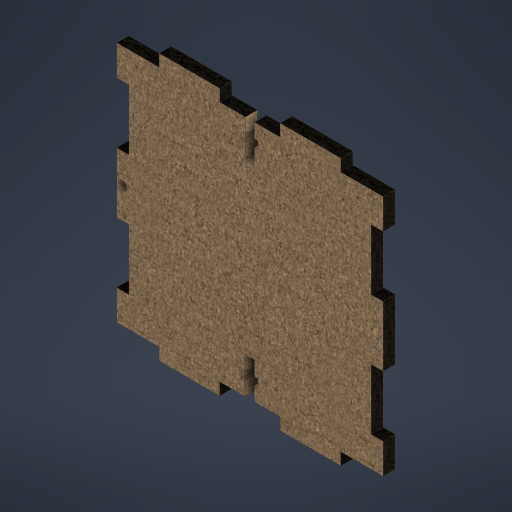
# Autodesk Inventor part: Car_Rear
Saved by Autodesk Inventor 2024.1 (Build 281209000, 209)
## iProperties
Created: 2023-08-04
Part Number: Car_Rear
Material: MDF Medium Density Fiberboard
Document SubType Name: Modeling
Designer: jaege
Density: 0.8 g/cm^3
Appearance: Cardboard - Corrugated
Author: jaege
Autodesk Inventor part; units mm, degrees
ref_plane "YZ Plane" through (0, 0, 0) normal (1, 0, 0) x (0, 1, 0)
ref_plane "XZ Plane" through (0, 0, 0) normal (0, 1, 0) x (-1, 0, 0)
ref_plane "XY Plane" through (0, 0, 0) normal (0, 0, 1) x (1, 0, 0)
sketch "Sketch1" plane through (0, 0, 0) normal (0, 0, 1) x (1, 0, 0)
  line L0 (70, 0) -> (80, 0) construction
  line L1 (80, 0) -> (80, 4) projected
  line L2 (70, 4) -> (80, 4) projected
  line L3 (70, 0) -> (70, 4) projected
  line L4 (50, 0) -> (70, 0) projected
  line L5 (30, 0) -> (50, 0) construction
  line L6 (50, 0) -> (50, 4) projected
  line L7 (30, 4) -> (50, 4) projected
  line L8 (30, 0) -> (30, 4) projected
  line L9 (10, 0) -> (30, 0) construction
  line L10 (0, -30) -> (0, -10) construction
  line L11 (0, -10) -> (-4, -10) projected
  line L12 (-4, -30) -> (-4, -10) projected
  line L13 (0, -30) -> (-4, -30) projected
  line L14 (0, -70) -> (0, -50) construction
  line L15 (0, -50) -> (-4, -50) projected
  line L16 (-4, -70) -> (-4, -50) projected
  line L17 (0, -70) -> (-4, -70) projected
  line L18 (0, -84) -> (10, -84) projected
  line L19 (10, -84) -> (10, -80) projected
  line L20 (0, -80) -> (10, -80) construction
  line L21 (0, -84) -> (0, -80) projected
  line L22 (10, -80) -> (30, -80) projected
  line L23 (30, -84) -> (50, -84) projected
  line L24 (50, -84) -> (50, -80) projected
  line L25 (30, -80) -> (50, -80) construction
  line L26 (30, -84) -> (30, -80) projected
  line L27 (50, -80) -> (70, -80) projected
  line L28 (70, -84) -> (80, -84) projected
  line L29 (80, -84) -> (80, -80) projected
  line L30 (70, -80) -> (80, -80) construction
  line L31 (70, -84) -> (70, -80) projected
  line L32 (0, 0) -> (0, -10)
  line L33 (0, 0) -> (10, 0) construction
  line L34 (10, 0) -> (10, 4) projected
  line L35 (0, 4) -> (10, 4) projected
  line L36 (0, 0) -> (0, 4) projected
  line L37 (0, -30) -> (0, -50)
  line L38 (0, -70) -> (0, -80)
  line L39 (0, 0) -> (80, -80) construction
  line L40 (40, -40) -> (40, 0) construction
  line L41 (80, -10) -> (84, -10)
  line L42 (84, -30) -> (84, -10)
  line L43 (80, -30) -> (84, -30)
  line L44 (80, -50) -> (84, -50)
  line L45 (84, -70) -> (84, -50)
  line L46 (80, -70) -> (84, -70)
  line L47 (80, 0) -> (80, -10)
  line L48 (80, -30) -> (80, -50)
  line L49 (80, -70) -> (80, -80)
  line L50 (0, -10) -> (-4, -10)
  line L51 (-4, -10) -> (-4, -30)
  line L52 (-4, -30) -> (0, -30)
  line L53 (0, -50) -> (-4, -50)
  line L54 (-4, -50) -> (-4, -70)
  line L55 (0, -70) -> (-4, -70)
  line L56 (0, -80) -> (0, -84)
  line L57 (0, -84) -> (10, -84)
  line L58 (10, -84) -> (10, -80)
  line L59 (10, -80) -> (30, -80)
  line L60 (30, -80) -> (30, -84)
  line L61 (50, -84) -> (30, -84)
  line L62 (50, -80) -> (50, -84)
  line L63 (50, -80) -> (70, -80)
  line L64 (70, -84) -> (70, -80)
  line L65 (70, -84) -> (80, -84)
  line L66 (80, -84) -> (80, -80)
  line L67 (80, 0) -> (80, 4)
  line L68 (0, 0) -> (0, 4)
  line L69 (10, 4) -> (0, 4)
  line L70 (10, 4) -> (10, 0)
  line L71 (10, 0) -> (30, 0)
  line L72 (30, 4) -> (30, 0)
  line L73 (30, 4) -> (50, 4)
  line L74 (50, 0) -> (50, 4)
  line L75 (50, 0) -> (70, 0)
  line L76 (70, 0) -> (70, 4)
  line L77 (70, 4) -> (80, 4)
  constraints: 84 end point, 15 collinear, 12 perpendicular, 8 symmetric about line, 2 midpoint, 2 parallel, 2 vertical
extrude "Extrusion1" add sketch "Sketch1" along normal blind 4
sketch "Sketch2" plane through (0, 0, 4) normal (0, 0, 1) x (1, 0, 0)
  line L0 (0, -10) -> (-4, -10) construction
  line L1 (-4, -10) -> (-4, -30) construction
  line L2 (-4, -30) -> (0, -30) construction
  line L3 (0, -30) -> (0, -50) construction
  line L4 (0, -50) -> (-4, -50) construction
  line L5 (-4, -50) -> (-4, -70) construction
  line L6 (-4, -70) -> (0, -70) construction
  line L7 (0, -70) -> (0, -84) construction
  line L8 (0, -84) -> (10, -84) construction
  line L9 (10, -84) -> (10, -80) construction
  line L10 (10, -80) -> (30, -80) construction
  line L11 (30, -80) -> (30, -84) construction
  line L12 (30, -84) -> (50, -84) construction
  line L13 (50, -84) -> (50, -80) construction
  line L14 (50, -80) -> (70, -80) construction
  line L15 (70, -80) -> (70, -84) construction
  line L16 (70, -84) -> (80, -84) construction
  line L17 (80, -84) -> (80, -70) construction
  line L18 (80, -70) -> (84, -70) construction
  line L19 (84, -70) -> (84, -50) construction
  line L20 (84, -50) -> (80, -50) construction
  line L21 (80, -50) -> (80, -30) construction
  line L22 (80, -30) -> (84, -30) construction
  line L23 (84, -30) -> (84, -10) construction
  line L24 (84, -10) -> (80, -10) construction
  line L25 (80, -10) -> (80, 4) construction
  line L26 (80, 4) -> (70, 4) construction
  line L27 (70, 4) -> (70, 0) construction
  line L28 (70, 0) -> (50, 0) construction
  line L29 (50, 0) -> (50, 4) construction
  line L30 (50, 4) -> (30, 4) construction
  line L31 (30, 4) -> (30, 0) construction
  line L32 (30, 0) -> (10, 0) construction
  line L33 (10, 0) -> (10, 4) construction
  line L34 (10, 4) -> (0, 4) construction
  line L35 (0, 4) -> (0, -10) construction
  circle A0 centre (40, 2) radius 1.5
  circle A1 centre (40, -82) radius 1.5
  line L36 (0, -38.5) -> (12, -38.5)
  line L37 (12, -38.5) -> (12, -41.5)
  line L38 (12, -41.5) -> (0, -41.5)
  line L39 (0, -41.5) -> (0, -38.5)
  line L40 (80, -38.5) -> (68, -38.5)
  line L41 (68, -38.5) -> (68, -41.5)
  line L42 (68, -41.5) -> (80, -41.5)
  line L43 (80, -41.5) -> (80, -38.5)
  line L44 (72.8, -42.7) -> (75.2, -42.7)
  line L45 (75.2, -42.7) -> (75.2, -37.3)
  line L46 (75.2, -37.3) -> (72.8, -37.3)
  line L47 (72.8, -37.3) -> (72.8, -42.7)
  line L48 (7.2, -42.7) -> (4.8, -42.7)
  line L49 (4.8, -42.7) -> (4.8, -37.3)
  line L50 (4.8, -37.3) -> (7.2, -37.3)
  line L51 (7.2, -37.3) -> (7.2, -42.7)
  line L52 (50, 0) -> (50, 4) construction
  line L53 (30, 0) -> (50, 4) construction
  line L54 (30, -84) -> (50, -80) construction
  point P0 (0, 0)
  point P1 (74, -37.3)
  point P2 (74, -38.5)
  point P3 (6, -37.3)
  point P4 (6, -38.5)
  point P5 (68, -40)
  point P6 (12, -40)
  point P7 (72.8, -40)
  point P8 (80, -40)
  point P9 (7.2, -38.5)
  point P10 (7.2, -41.5)
  point P11 (72.8, -38.5)
  point P12 (72.8, -41.5)
  point P13 (4.8, -41.5)
  point P14 (4.8, -38.5)
  point P15 (75.2, -38.5)
  point P16 (75.2, -41.5)
  dimension "d2" = 3
  dimension "d3" = 2.4
  dimension "d4" = 5.4
  dimension "d5" = 3
  dimension "d6" = 12
  constraints: 36 end point, 10 midpoint, 8 parallel, 5 horizontal alignment, 4 horizontal, 4 perpendicular, 4 point on line, 2 centre point, 2 collinear, 2 vertical alignment, 1 equal radius
  measures "d2" diameter of A0
  measures "d3" distance of L49.end L50.end
  measures "d4" distance of L50.end L48.start
  measures "d5" distance of L36.end L37.end
  measures "d6" distance of L36.start L36.end
extrude "Extrusion2" cut sketch "Sketch2" against normal up to next
body "Solid1"
